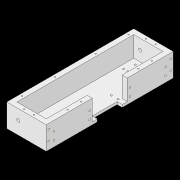
# Autodesk Inventor part: AfterComp1Chassis
Saved by Autodesk Inventor 2021 (Build 250183000, 183)
## iProperties
Created: 2021-02-15
Part Number: AfterComp1Chassis
Material: UHMW, White
Document SubType Name: Modeling
Designer: Esketitttttt
Density: 0.94 g/cm^3
Appearance: Smooth - White
Mass: 73.8354 g
Surface Area: 364.172 cm^2
Volume: 78.5483 cm^3
Author: Esketitttttt
Autodesk Inventor part; units mm, degrees
ref_plane "YZ Plane" through (0, 0, 0) normal (1, 0, 0) x (0, 1, 0)
ref_plane "XZ Plane" through (0, 0, 0) normal (0, 1, 0) x (-1, 0, 0)
sketch "BasePlan" plane through (0, 0, 0) normal (0, 1, 0) x (-1, 0, 0)
  line L0 (0, 0) -> (-36.42, 0)
  line L1 (-36.42, 0) -> (-36.42, -30.9122)
  line L2 (-36.42, -30.9122) -> (0, -30.9122)
  line L3 (0, -30.9122) -> (0, 0)
  line L4 (0, 0) -> (-16.1, 0)
  line L5 (-16.1, 0) -> (-16.1, 57.15)
  line L6 (-16.1, 57.15) -> (0, 57.15)
  line L7 (0, 57.15) -> (0, 0)
  line L8 (-16.1, 57.15) -> (-36.42, 57.15)
  line L9 (-36.42, 57.15) -> (-36.42, 0)
  line L10 (-36.42, 0) -> (-16.1, 0)
  line L11 (-16.1, 0) -> (-16.1, 57.15)
  line L12 (0, 0) -> (0, -15.4561)
  line L13 (0, -15.4561) -> (8.9825, -15.4561) construction
  line L14 (-16.1, -30.9122) -> (-16.1, -88.0622)
  line L15 (-16.1, -88.0622) -> (0, -88.0622)
  line L16 (0, -88.0622) -> (0, -30.9122)
  line L17 (-16.1, -88.0622) -> (-36.42, -88.0622)
  line L18 (-36.42, -88.0622) -> (-36.42, -30.9122)
  line L19 (0, -88.0622) -> (6.35, -88.0622) construction
  line L20 (6.35, -88.0622) -> (6.35, -94.4122) construction
  line L21 (6.35, -94.4122) -> (0, -94.4122) construction
  line L22 (0, -94.4122) -> (0, -88.0622) construction
  line L23 (0, 57.15) -> (6.35, 57.15) construction
  line L24 (6.35, 57.15) -> (6.35, 63.5) construction
  line L25 (6.35, 63.5) -> (0, 63.5) construction
  line L26 (0, 63.5) -> (0, 57.15) construction
  line L27 (-36.42, -88.0622) -> (-42.77, -88.0622) construction
  line L28 (-42.77, -88.0622) -> (-42.77, -94.4122) construction
  line L29 (-42.77, -94.4122) -> (-36.42, -94.4122) construction
  line L30 (-36.42, -94.4122) -> (-36.42, -88.0622) construction
  line L31 (-36.42, 57.15) -> (-42.77, 57.15) construction
  line L32 (-42.77, 57.15) -> (-42.77, 63.5) construction
  line L33 (-42.77, 63.5) -> (-36.42, 63.5) construction
  line L34 (-36.42, 63.5) -> (-36.42, 57.15) construction
  line L35 (-42.77, 63.5) -> (-36.42, 63.5)
  line L36 (-36.42, 63.5) -> (-36.42, 0)
  line L37 (-36.42, 0) -> (-42.77, 0)
  line L38 (-42.77, 0) -> (-42.77, 63.5)
  line L39 (6.35, 63.5) -> (0, 63.5)
  line L40 (0, 63.5) -> (0, -94.4122)
  line L41 (0, -94.4122) -> (6.35, -94.4122)
  line L42 (6.35, -94.4122) -> (6.35, 63.5)
  line L43 (-36.42, 63.5) -> (0, 63.5)
  line L44 (0, 63.5) -> (0, 57.15)
  line L45 (0, 57.15) -> (-36.42, 57.15)
  line L46 (-36.42, 57.15) -> (-36.42, 63.5)
  line L47 (-36.42, -88.0622) -> (0, -88.0622)
  line L48 (0, -88.0622) -> (0, -94.4122)
  line L49 (0, -94.4122) -> (-36.42, -94.4122)
  line L50 (-36.42, -94.4122) -> (-36.42, -88.0622)
  line L51 (-42.77, -94.4122) -> (-36.42, -94.4122)
  line L52 (-36.42, -94.4122) -> (-36.42, -30.9122)
  line L53 (-36.42, -30.9122) -> (-42.77, -30.9122)
  line L54 (-42.77, -30.9122) -> (-42.77, -94.4122)
  line L55 (-36.42, -30.9122) -> (-42.77, -30.9122)
  line L56 (-42.77, -30.9122) -> (-42.77, -37.2622)
  line L57 (-42.77, -37.2622) -> (-36.42, -37.2622)
  line L58 (-36.42, -37.2622) -> (-36.42, -30.9122)
  line L59 (-36.42, 0) -> (-42.77, 0)
  line L60 (-42.77, 0) -> (-42.77, 6.35)
  line L61 (-42.77, 6.35) -> (-36.42, 6.35)
  line L62 (-36.42, 6.35) -> (-36.42, 0)
  point P0 (-36.42, 6.35)
  dimension "d3" = 16.1
  dimension "d5" = 20.32
  dimension "d6" = 30.9122
  dimension "d7" = 57.15
  dimension "d8" = 36.42
  dimension "d9" = 36.42
  dimension "d10" = 15.4561
  dimension "d12" = 6.35
  dimension "d88" = 6.35
  dimension "d89" = 6.35
  dimension "d90" = 6.35
  dimension "d158" = 157.9122
  constraints: 126 end point, 28 parallel, 15 horizontal, 14 perpendicular, 7 equal length, 5 symmetric about line, 2 point on line, 1 midpoint
  measures "d3" distance of L5.end L6.end
  measures "d5" distance of L5.end L8.end
  measures "d6" distance of L2.end L0.start
  measures "d7" distance of L6.end L0.start
  measures "d8" distance of L8.end L6.end
  measures "d9" distance of L1.end L2.end
  measures "d10" distance of L0.start L12.end
  measures "d12" distance of L19.end L20.end
  measures "d88" distance of L57.end L56.end
  measures "d89" distance of L56.end L55.end
  measures "d90" distance of L59.end L60.end
  measures "d158" distance of L41.end L24.end
extrude "BackWall" add sketch "BasePlan" along normal blind 25.4 contours L7 L40 L39 L42 L41 L16 L3
sketch "Sketch2" plane through (-6.35, 0, -94.4122) normal (-1, 0, 0) x (0, 0, 1)
  line L0 (0, 0) -> (0, 25.4) construction
  line L1 (0, 0) -> (157.9122, 0) construction
  line L2 (0, 0) -> (3.175, 0) construction
  line L3 (3.175, 0) -> (3.175, 6.35) construction
  line L4 (3.175, 6.35) -> (0, 6.35) construction
  line L5 (0, 6.35) -> (0, 0) construction
  line L6 (3.175, 0) -> (3.175, 19.05) construction
  line L7 (0, 25.4) -> (157.9122, 25.4) projected
  line L8 (0, 25.4) -> (78.9561, 25.4) construction
  line L9 (78.9561, 25.4) -> (78.9561, 53.975) construction
  point P0 (94.4122, 0)
  point P1 (6.35, 0)
  point P2 (154.7372, 19.05)
  point P3 (154.7372, 6.35)
  dimension "d25" = 6.35
  dimension "d26" = 25.4
  dimension "d27" = 3.175
  dimension "d28" = 6.35
  dimension "d29" = 19.05
  dimension "d30" = 157.9122
  dimension "d31" = 78.9561
  constraints: 14 end point, 2 coincident, 2 parallel, 2 symmetric about line, 1 horizontal, 1 midpoint, 1 perpendicular, 1 point on line, 1 vertical
  measures "d25" distance of L0.start point (6.35, 0)
  measures "d26" distance of L0.start L0.end
  measures "d27" distance of L4.end L3.end
  measures "d28" distance of L3.end L2.end
  measures "d29" distance of L2.end L6.end
  measures "d30" distance of L0.end L7.end
  measures "d31" distance of L0.end L8.end
extrude "LeftSideWall" add sketch "BasePlan" along normal up to surface (25.4 mm away) contours L40 L49 L50 L17 L15
extrude "RightSideWall" add sketch "BasePlan" along normal up to surface (25.4 mm away) contours L6 L8 L36 L43 L40
hole "BackHoles" at (-6.35, 6.35, -91.2372) at (-6.35, 19.05, -91.2372) at (-6.35, 19.05, 60.325) at (-6.35, 6.35, 60.325) direction (1, 0, 0) diameter 1.524 depth 9.525 tip angle 118
extrude "RightFrontWall" add sketch "BasePlan" along normal up to surface (25.4 mm away) contours L61 L38 L35 L36 L9
extrude "LeftFrontWall" add sketch "BasePlan" along normal up to surface (25.4 mm away) contours L18 L50 L51 L54 L57
extrude "BottomUHMW" add sketch "BasePlan" against normal blind 3.175
sketch "Sketch4" plane through (0, -3.175, 0) normal (0, -1, 0) x (1, 0, 0)
  line L0 (-4.7625, -65.2173) -> (-4.7625, -63.6933) construction
  line L1 (-4.7625, -65.2173) -> (-4.7625, -63.6933) construction
  line L2 (0, -94.4122) -> (0, -88.0622) construction
  line L3 (-6.35, -88.5497) -> (-6.35, -94.4122) construction
  line L4 (-6.35, -83.7872) -> (-6.35, -88.5497) construction
  line L5 (0, 50.8) -> (0, -88.0622)
  line L6 (0, -18.6311) -> (-6.35, -18.6311)
  line L7 (39.595, -37.2622) -> (42.77, -37.2622) construction
  line L8 (42.77, -37.2622) -> (42.77, -54.1955) construction
  line L9 (42.77, -54.1955) -> (39.595, -54.1955) construction
  line L10 (39.595, -54.1955) -> (39.595, -37.2622) construction
  line L11 (39.595, -75.8914) -> (39.595, -71.1289) construction
  line L12 (-6.35, -94.4122) -> (42.77, -94.4122) projected
  line L13 (-6.35, -94.4122) -> (42.77, -94.4122) projected
  line L14 (-6.35, -94.4122) -> (-3.175, -94.4122)
  line L15 (-3.175, -94.4122) -> (-3.175, -84.8872) construction
  line L16 (36.42, -88.0622) -> (0, -88.0622) projected
  line L17 (-3.175, -94.4122) -> (-3.175, -43.8915) construction
  line L18 (42.77, -94.4122) -> (42.77, -30.9122) projected
  line L19 (42.77, -37.2622) -> (36.42, -37.2622) projected
  point P0 (0, 0)
  point P1 (-7.579, 35.8142)
  point P2 (-3.175, 47.625)
  point P3 (-3.175, 6.6293)
  point P4 (42.77, 16.9333)
  point P5 (39.595, 33.8667)
  point P6 (39.595, 16.9333)
  dimension "d91" = 3.175
  dimension "d104" = 4.7625
  dimension "d118" = 3.175
  dimension "d119" = 9.525
  dimension "d121" = 75.7811
  dimension "d132" = 50.5207
  dimension "d160" = 50.8
  dimension "d161" = 16.9333
  dimension "d162" = 16.9333
  dimension "d195" = 0
  constraints: 30 end point, 6 coincident, 5 symmetric about line, 4 point on line, 2 midpoint, 2 parallel, 2 perpendicular, 1 horizontal, 1 vertical
  measures "d91" distance of L8.end L9.end
  measures "d104" distance of L11.start L11.end
  measures "d118" distance of L3.end L14.end
  measures "d119" distance of L14.end L15.end
  measures "d121" distance between parallel lines of L12 L6
  measures "d132" distance of L14.end L17.end
  measures "d160" vertical distance of L16.start L19.start
  measures "d161" vertical distance of point (39.595, -71.129) L16.start
  measures "d162" distance of point (42.77, -54.196) L19.start
  measures "d195" distance between parallel lines of L10 L11
hole "BottomHoles" at (-3.175, -3.175, 47.625) at (-3.175, -3.175, -84.8872) at (39.595, -3.175, -71.1289) at (-3.175, -3.175, -43.8915) at (-3.175, -3.175, 6.6293) at (39.595, -3.175, 33.8667) at (39.595, -3.175, -54.1955) at (39.595, -3.175, 16.9333) direction (0, 1, 0) diameter 1.524 depth 9.525 tip angle 118
sketch "Sketch5" plane through (0, 25.4, 0) normal (0, 1, 0) x (1, 0, 0)
  line L0 (-6.35, -63.5) -> (-1.5875, -63.5) construction
  line L1 (-1.5875, -63.5) -> (-1.5875, -58.7375) construction
  line L2 (-1.5875, -58.7375) -> (-6.35, -58.7375) construction
  line L3 (-6.35, -58.7375) -> (-6.35, -63.5) construction
  line L4 (-6.35, -58.7375) -> (-3.9687, -58.7375) construction
  line L5 (-3.9687, -58.7375) -> (-3.9687, -53.975) construction
  line L6 (-3.9687, -53.975) -> (-6.35, -53.975) construction
  line L7 (-6.35, -53.975) -> (-6.35, -58.7375) construction
  line L8 (23.9254, -63.0415) -> (25.7232, -67.4516)
  line L9 (20.7687, 15.4561) -> (-4.7625, 15.4561)
  line L10 (-6.35, -63.5) -> (42.77, -63.5) projected
  line L11 (-6.35, 94.4122) -> (-6.35, -63.5) projected
  line L12 (-6.35, 15.4561) -> (-15.875, 15.4561)
  line L13 (37.5312, -37.0575) -> (37.5312, -32.295) construction
  line L14 (-59.5503, 62.2293) -> (-59.5503, 57.4668) construction
  circle A0 centre (39.595, 71.1289) radius 0.762 projected
  circle A1 centre (38.8013, -32.295) radius 1.0922 projected
  point P0 (0, 0)
  point P1 (-3.9687, 84.8872)
  point P2 (-3.9687, 84.8872)
  dimension "d63" = 17.7775
  dimension "d64" = 2.3813
  dimension "d65" = 4.7625
  dimension "d66" = 0
  dimension "d106" = 4.7625
  dimension "d107" = 4.7625
  constraints: 26 end point, 6 symmetric about line, 4 coincident, 4 parallel, 3 horizontal, 2 perpendicular, 2 vertical, 2 other
  measures "d64" distance of L6.end L5.end
  measures "d65" distance of L5.end L4.end
  measures "d66" distance between parallel lines of L12 L9
  measures "d106" distance of L13.start L13.end
  measures "d107" distance of L14.start L14.end
hole "TopHoles" [suppressed]
sketch "Sketch6" plane through (42.77, 1.5875, 96.9182) normal (1, 0, 0) x (0, 0, -1)
  line L0 (33.4183, -1.5999) -> (33.4183, 23.8001) construction
  line L1 (0, 0) -> (146.8373, -1.5875) construction
  line L2 (33.4183, -1.5999) -> (36.5933, -1.5999) construction
  line L3 (36.5933, -1.5999) -> (36.5933, 4.7501) construction
  line L4 (36.5933, 4.7501) -> (33.4183, 4.7501) construction
  line L5 (33.4183, 4.7501) -> (33.4183, -1.5999) construction
  line L6 (36.5933, -1.5999) -> (36.5933, 17.4501) construction
  line L7 (33.4183, 23.8001) -> (191.3304, 23.8125)
  line L8 (0, 25.4) -> (57.8525, 25.4) construction
  line L9 (57.8525, 25.4) -> (57.8525, 53.975) construction
  line L10 (112.3743, 23.8063) -> (112.3743, 30.1563)
  line L11 (191.3304, -4.7625) -> (191.3304, 23.8125) projected
  line L12 (33.4182, 23.8125) -> (33.4182, -4.7625) projected
  point P0 (66.8365, 0)
  point P1 (39.7651, -1.4015)
  point P2 (146.8372, -1.5875)
  point P3 (0, 0)
  point P4 (188.1554, 17.4501)
  point P5 (188.1554, 4.7501)
  dimension "d85" = 6.35
  dimension "d86" = 25.4
  dimension "d77" = 3.175
  dimension "d78" = 6.35
  dimension "d76" = 19.05
  dimension "d87" = 157.9122
  dimension "d75" = 57.8525
  dimension "d164" = 157.9122
  constraints: 20 end point, 3 vertical, 2 coincident, 2 parallel, 2 symmetric about line, 1 horizontal, 1 midpoint, 1 perpendicular, 1 point on line, 3 other
  measures "d85" distance of L0.start point (39.765, -1.401)
  measures "d86" distance of L0.start L0.end
  measures "d77" distance of L4.end L3.end
  measures "d78" distance of L3.end L2.end
  measures "d76" distance of L2.end L6.end
  measures "d87" distance of L0.end L7.end
  measures "d75" distance of L8.start L8.end
  measures "d164" distance between parallel lines of L11 L12
hole "Front Holes" at (42.77, 6.3376, 60.325) at (42.77, 19.0376, 60.325) at (42.77, 19.0376, -91.2372) at (42.77, 6.3376, -91.2372) direction (-1, 0, 0) diameter 2.1844 depth 9.525 tip angle 118
sketch "Sketch7" plane through (36.42, 25.4, 57.15) normal (0, 0, -1) x (-1, 0, 0)
  line L0 (28.3682, -22.225) -> (28.3682, -12.7) construction
  line L1 (28.3682, -12.7) -> (36.42, -12.7) construction
  line L2 (36.42, -12.7) -> (36.42, -25.4)
  circle A0 centre (28.3682, -12.7) radius 8.04 construction
  circle A1 centre (28.3682, -12.7) radius 2.96
  line L3 (28.3682, -12.7) -> (28.3682, -7.2) construction
  line L4 (28.3682, -12.7) -> (28.3682, -18.2) construction
  circle A2 centre (28.3682, -18.2) radius 1.143
  circle A3 centre (28.3682, -7.2) radius 1.143
  circle A4 centre (28.3682, -12.7) radius 2
  line L5 (35.15, -9.525) -> (27.11, -9.525) construction
  line L6 (36.42, 0) -> (36.42, -25.4) projected
  dimension "d93" = 8.0518
  dimension "d94" = 5.5
  dimension "d95" = 5.5
  dimension "d96" = 2.286
  dimension "d97" = 2.286
  dimension "d98" = 4
  dimension "d101" = 12.7
  dimension "d194" = 0
  constraints: 12 end point, 5 centre point, 5 coincident, 1 horizontal, 1 parallel, 1 vertical
  measures "d93" distance of L3.start L1.end
  measures "d94" distance of L3.start L3.end
  measures "d95" distance of L3.start L4.end
  measures "d96" diameter of A2
  measures "d97" diameter of A3
  measures "d98" diameter of A4
  measures "d101" distance of L1.end L2.end
  measures "d194" distance between parallel lines of L2 L6
extrude "MotorHole" cut sketch "Sketch7" along normal through all both and the other way through all contours A4
sketch "Sketch8" plane through (0, -3.175, 0) normal (0, -1, 0) x (1, 0, 0)
  line L0 (39.9125, -21.354) -> (16.238, -21.354)
  line L1 (17.8251, -30.9122) -> (17.8251, -37.2622)
  line L2 (17.8251, -34.0872) -> (26.1401, -34.0872) construction
  line L3 (26.1401, -34.0872) -> (34.455, -34.0872) construction
  line L4 (36.42, -30.9122) -> (36.42, 0) projected
  line L5 (36.42, -15.4561) -> (39.9125, -15.4561)
  line L6 (17.8251, 3.175) -> (26.1401, 3.175) construction
  line L7 (26.1401, 3.175) -> (34.455, 3.175) construction
  line L8 (42.77, -37.2622) -> (36.42, -37.2622) projected
  line L9 (17.8251, -37.2622) -> (42.77, -37.2622)
  point P0 (0, 0)
  point P1 (0, 44.9224)
  point P2 (16.238, -21.354)
  point P3 (42.77, -30.9122)
  dimension "d109" = 8.315
  dimension "d110" = 8.315
  dimension "d196" = 3.175
  dimension "d197" = 3.175
  dimension "d198" = 3.175
  constraints: 14 end point, 5 symmetric about line, 4 coincident, 2 midpoint, 1 collinear, 1 horizontal, 3 other
  measures "d109" distance of L2.start L2.end
  measures "d110" distance of L2.end L3.end
  measures "d196" distance from line of L9 L3.end
  measures "d197" distance from line of point (26.14, -34.087) L9
  measures "d198" distance of L1.end L2.start
hole "UprightHoles" at (26.1401, -3.175, -34.0872) at (34.455, -3.175, -34.0872) at (34.455, -3.175, 3.175) at (26.1401, -3.175, 3.175) direction (0, 1, 0) diameter 2.1844 depth 9.525 tip angle 118
sketch "Sketch9" plane through (0, -3.175, 0) normal (0, -1, 0) x (1, 0, 0)
  line L0 (0, 57.15) -> (36.42, 57.15) construction
  line L1 (36.42, -88.0622) -> (0, -88.0622) construction
  line L2 (-6.35, -94.4122) -> (42.77, -94.4122) construction
  line L3 (-6.35, 63.5) -> (42.77, 63.5) construction
  line L4 (36.42, 57.15) -> (36.42, 6.35) construction
  line L5 (36.42, -37.2622) -> (36.42, -88.0622) construction
  line L6 (0, 57.15) -> (0, -88.0622) construction
  line L7 (0, -88.0622) -> (36.42, -88.0622) construction
  line L8 (36.42, -88.0622) -> (36.42, -94.4122) construction
  line L9 (-6.35, -94.4122) -> (42.77, -94.4122) construction
  line L10 (0, -88.0622) -> (0, -94.4122) construction
  line L11 (0, 57.15) -> (0, 63.5) construction
  line L12 (42.77, 63.5) -> (-6.35, 63.5) construction
  line L13 (36.42, 57.15) -> (36.42, 63.5) construction
  line L14 (36.42, -91.2372) -> (24.28, -91.2372) construction
  line L15 (24.28, -91.2372) -> (12.14, -91.2372) construction
  line L16 (0, -15.4561) -> (7.9375, -15.4561)
  line L17 (-6.35, 63.5) -> (-6.35, -94.4122) projected
  point P0 (0, 0)
  point P1 (12.14, 60.325)
  point P2 (24.28, 60.325)
  dimension "d122" = 36.42
  dimension "d123" = 12.14
  dimension "d124" = 12.14
  dimension "d163" = 6.35
  constraints: 14 end point, 5 point on line, 3 perpendicular, 2 coincident, 2 horizontal, 2 midpoint, 2 symmetric about line, 1 parallel
  measures "d122" distance of L1.start L1.end
  measures "d123" distance of L14.start L14.end
  measures "d124" distance of L14.end L15.end
  measures "d163" distance from line of L17 L1.end
hole "SideWallBottomHoles" at (12.14, -3.175, -91.2372) at (24.28, -3.175, -91.2372) at (12.14, -3.175, 60.325) at (24.28, -3.175, 60.325) direction (0, 1, 0) diameter 1.524 depth 9.525 tip angle 118
ref_plane "MidHeightPlane" through (0, 11.1125, 0) normal (0, 1, 0) x (1, 0, 0)
mirror "Mirror1" about plane through (0, 11.1125, 0) normal (0, 1, 0) of "BottomHoles", "SideWallBottomHoles"
sketch "Sketch10" plane through (42.77, 25.4, 63.5) normal (1, 0, 0) x (0, 0, -1)
  circle A0 centre (9.525, -21.4312) radius 1.0922
  circle A1 centre (9.525, -11.9062) radius 1.0922
  circle A2 centre (53.975, -11.9062) radius 1.0922
  circle A3 centre (53.975, -21.4312) radius 1.0922
  circle A4 centre (103.9372, -21.4312) radius 1.0922
  circle A5 centre (103.9372, -11.9062) radius 1.0922
  circle A6 centre (148.3872, -11.9062) radius 1.0922
  circle A7 centre (148.3872, -21.4312) radius 1.0922
  line L0 (41.82, 0) -> (0, 0)
  line L1 (114.519, 0) -> (72.699, 0)
  line L2 (57.15, 0) -> (0, 0) projected
  line L3 (0, 0) -> (0, -28.575) projected
  line L4 (57.15, -25.4) -> (57.15, 0) projected
  line L5 (100.7622, -25.4) -> (100.7622, 0) projected
  line L6 (157.9122, -28.575) -> (157.9122, 0) projected
  line L7 (157.9122, 0) -> (100.7622, 0) projected
  dimension "d167" = 9.525
  dimension "d168" = 9.525
  dimension "d169" = 3.175
  dimension "d170" = 3.175
  dimension "d171" = 9.525
  dimension "d172" = 9.525
  dimension "d173" = 3.175
  dimension "d174" = 3.175
  dimension "d175" = 9.525
  dimension "d176" = 9.525
  dimension "d177" = 9.525
  dimension "d178" = 11.9062
  dimension "d179" = 11.9062
  dimension "d180" = 2.1844
  dimension "d181" = 2.1844
  dimension "d182" = 2.1844
  dimension "d183" = 2.1844
  dimension "d184" = 2.1844
  dimension "d185" = 2.1844
  dimension "d186" = 2.1844
  dimension "d187" = 2.1844
  constraints: 8 centre point, 4 end point
  measures "d167" distance from line of L3 A1.centre
  measures "d168" distance from line of L3 A0.centre
  measures "d169" distance from line of A2.centre L4
  measures "d170" distance from line of L4 A3.centre
  measures "d171" distance of A3.centre A2.centre
  measures "d172" distance of A0.centre A1.centre
  measures "d173" distance from line of A5.centre L5
  measures "d174" distance from line of L5 A4.centre
  measures "d175" distance from line of A6.centre L6
  measures "d176" distance from line of L6 A7.centre
  measures "d177" distance of A7.centre A6.centre
  measures "d178" distance from line of L2 A1.centre
  measures "d179" distance from line of L7 A6.centre
  measures "d180" diameter of A7
  measures "d181" diameter of A6
  measures "d182" diameter of A5
  measures "d183" diameter of A4
  measures "d184" diameter of A3
  measures "d185" diameter of A2
  measures "d186" diameter of A0
  measures "d187" diameter of A1
hole "WedgeletHoles" at (42.77, 13.4938, 53.975) at (42.77, 3.9688, 53.975) at (42.77, 13.4938, 9.525) at (42.77, 3.9688, 9.525) at (42.77, 13.4938, -40.4372) at (42.77, 3.9688, -40.4372) at (42.77, 13.4938, -84.8872) at (42.77, 3.9688, -84.8872) direction (-1, 0, 0) diameter 2.1844 depth 9.525 tip angle 118
sketch "Sketch11" plane through (0, -3.175, 0) normal (0, -1, 0) x (1, 0, 0)
  line L0 (-6.35, -94.4122) -> (-6.35, 63.5) projected
  line L1 (42.77, -94.4122) -> (42.77, -37.2622) projected
  line L2 (-6.35, 63.5) -> (42.77, 63.5)
  line L3 (42.77, 63.5) -> (42.77, -94.4122)
  line L4 (42.77, -94.4122) -> (-6.35, -94.4122)
  line L5 (-6.35, -94.4122) -> (-6.35, 63.5)
  line L6 (36.42, -88.0622) -> (36.42, 57.15)
  line L7 (36.42, 57.15) -> (0, 57.15)
  line L8 (0, 57.15) -> (0, -88.0622)
  line L9 (0, -88.0622) -> (36.42, -88.0622)
  line L10 (16.08, 33.15) -> (0, 33.15) construction
  line L11 (0, 33.15) -> (0, 57.15)
  line L12 (16.08, 33.15) -> (16.08, 45.15)
  line L13 (16.08, 45.15) -> (0, 45.15)
  line L14 (0, 45.15) -> (0, 33.15)
  line L15 (0, 33.15) -> (16.08, 33.15) construction
  line L16 (16.08, 33.15) -> (16.08, 57.15)
  line L17 (16.08, 32.995) -> (16.08, 57.15)
  line L18 (0, 45.15) -> (16.08, 57.15)
  line L19 (16.08, 33.15) -> (16.08, 39.15)
  line L20 (16.08, 39.15) -> (10.72, 39.15)
  line L21 (10.72, 39.15) -> (10.72, 33.15)
  line L22 (10.72, 33.15) -> (16.08, 33.15)
  line L23 (10.72, 33.15) -> (10.72, 39.15)
  line L24 (10.72, 39.15) -> (5.36, 39.15)
  line L25 (5.36, 39.15) -> (5.36, 33.15)
  line L26 (5.36, 33.15) -> (10.72, 33.15)
  line L27 (16.08, 57.15) -> (0, 57.15)
  line L28 (36.42, 0) -> (36.42, -30.9122) projected
  line L29 (36.42, -15.4561) -> (17.145, -15.4561)
  line L30 (36.42, -15.4561) -> (55.695, -15.4561) construction
  point P0 (0, 0)
  point P1 (8.04, 51.15)
  point P2 (8.04, -82.0622)
  point P3 (5.36, -70.0622)
  point P4 (10.72, -70.0622)
  dimension "d140" = 6.35
  dimension "d144" = 12
  dimension "d146" = 6
  dimension "d147" = 5.36
  dimension "d148" = 6
  dimension "d149" = 5.36
  dimension "d150" = 180
  dimension "d189" = 0
  dimension "d190" = 0
  dimension "d192" = 12
  dimension "d193" = 5.36
  constraints: 54 end point, 9 parallel, 5 horizontal, 5 perpendicular, 4 midpoint, 3 coincident, 3 symmetric about line, 2 vertical, 1 collinear, 6 other
  measures "d140" distance between parallel lines of L3 L6
  measures "d144" distance of L12.end L16.start
  measures "d146" distance of L26.end L20.end
  measures "d147" distance of L20.end L20.start
  measures "d148" distance of L26.start L24.end
  measures "d149" distance of L24.end L24.start
  measures "d150" angle of L29 L30
  measures "d189" distance between parallel lines of L7 L27
  measures "d190" distance between parallel lines of L8 L11
  measures "d193" distance from line of L14 L24.end
hole "BottomMotorMountHoles" at (8.04, -3.175, 51.15) at (5.36, -3.175, 39.15) at (10.72, -3.175, 39.15) at (8.04, -3.175, -82.0622) at (5.36, -3.175, -70.0622) at (10.72, -3.175, -70.0622) direction (0, 1, 0) diameter 2.1844 depth 9.525 tip angle 118
sketch "FrontWallDrawing" plane through (42.77, 25.4, -37.2622) normal (1, 0, 0) x (0, 0, -1)
  line L0 (0, -25.4) -> (0, 0) projected
  circle A0 centre (3.175, -11.9062) radius 1.0922 projected
  circle A1 centre (3.175, -21.4312) radius 1.0922 projected
  circle A2 centre (47.625, -11.9062) radius 1.0922 projected
  circle A3 centre (47.625, -21.4312) radius 1.0922 projected
  line L1 (0, -25.4) -> (50.8, -25.4)
  line L2 (50.8, 0) -> (0, 0)
  line L3 (57.15, 0) -> (0, 0) projected
  line L4 (50.8, -25.4) -> (57.15, -25.4)
  line L5 (57.15, -25.4) -> (57.15, 0)
  circle A4 centre (53.975, -6.3624) radius 1.0922 projected
  circle A5 centre (53.975, -19.0624) radius 1.0922 projected
  point P0 (-37.2622, -25.4)
  constraints: 8 end point, 2 horizontal, 1 vertical
sketch "SideWallDrawing" plane through (42.77, 25.4, -94.4122) normal (0, 0, -1) x (-1, 0, 0)
  line L0 (42.77, -25.4) -> (6.35, -25.4) projected
  line L1 (6.35, 0) -> (42.77, 0) projected
  line L2 (42.77, -25.4) -> (42.77, 0) projected
  line L3 (6.35, -25.4) -> (6.35, 0) projected
  circle A0 centre (34.7182, -12.7) radius 2 projected
sketch "BackWallDrawing" plane through (-6.35, 25.4, -94.4122) normal (-1, 0, 0) x (0, 0, 1)
  line L0 (151.5622, -25.4) -> (6.35, -25.4) projected
  line L1 (0, 0) -> (157.9122, 0) projected
  line L2 (151.5622, -25.4) -> (157.9122, -25.4)
  line L3 (157.9122, -25.4) -> (157.9122, 0)
  line L4 (6.35, -25.4) -> (0, -25.4)
  line L5 (0, 0) -> (0, -25.4)
  circle A0 centre (154.7372, -6.35) radius 0.762 projected
  circle A1 centre (154.7372, -19.05) radius 0.762 projected
  circle A2 centre (3.175, -19.05) radius 0.762 projected
  circle A3 centre (3.175, -6.35) radius 0.762 projected
  point P0 (94.4122, -25.4)
  constraints: 8 end point, 1 horizontal
sketch "BottomPlateDrawing" plane through (0, -3.175, 0) normal (0, -1, 0) x (1, 0, 0)
  circle A0 centre (5.36, -70.0622) radius 1.0922 projected
  circle A1 centre (10.72, 39.15) radius 1.0922 projected
  circle A2 centre (8.04, 51.15) radius 1.0922 projected
  circle A3 centre (5.36, 39.15) radius 1.0922 projected
  circle A4 centre (8.04, -82.0622) radius 1.0922 projected
  circle A5 centre (10.72, -70.0622) radius 1.0922 projected
  circle A6 centre (12.14, 60.325) radius 0.762 projected
  circle A7 centre (12.14, -91.2372) radius 0.762 projected
  circle A8 centre (24.28, -91.2372) radius 0.762 projected
  circle A9 centre (24.28, 60.325) radius 0.762 projected
  circle A10 centre (34.455, 3.175) radius 1.0922 projected
  circle A11 centre (26.1401, -34.0872) radius 1.0922 projected
  circle A12 centre (34.455, -34.0872) radius 1.0922 projected
  circle A13 centre (26.1401, 3.175) radius 1.0922 projected
  circle A14 centre (-3.175, -43.8915) radius 0.762 projected
  circle A15 centre (-3.175, 47.625) radius 0.762 projected
  circle A16 centre (-3.175, -84.8872) radius 0.762 projected
  circle A17 centre (39.595, -71.1289) radius 0.762 projected
  circle A18 centre (-3.175, 6.6293) radius 0.762 projected
  circle A19 centre (39.595, 33.8667) radius 0.762 projected
  line L0 (42.77, -30.9122) -> (36.42, -30.9122) projected
  line L1 (36.42, -30.9122) -> (36.42, 0) projected
  line L2 (36.42, 0) -> (42.77, 0) projected
  line L3 (42.77, 63.5) -> (-6.35, 63.5) projected
  line L4 (-6.35, 63.5) -> (-6.35, -94.4122) projected
  line L5 (-6.35, -94.4122) -> (42.77, -94.4122) projected
  line L6 (42.77, -94.4122) -> (42.77, -30.9122) projected
  line L7 (42.77, 0) -> (42.77, 63.5) projected
  point P0 (0, 0)
equation "\"d9\" = d8"
equation "\"d10\" = 0.5 * d6"
equation "\"d27\" = 0.5 * d25"
equation "\"d28\" = 0.25 * d26"
equation "\"d29\" = 3 * d28"
equation "\"d31\" = 0.5 * d30"
equation "\"d121\" = 0.5 * d120"
equation "\"d132\" = 0.333333 * d120"
equation "\"d77\" = 0.5 * d85"
equation "\"d78\" = 0.25 * d86"
equation "\"d76\" = 3 * d78"
equation "\"d123\" = 0.333333 * d122"
equation "\"d124\" = 0.333333 * d122"
equation "\"d149\" = d147"
equation "\"d120\" = 151.56219"
body "Solid1"
